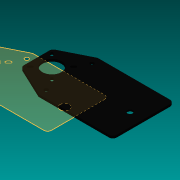
# Autodesk Inventor part: Y Slider
Saved by Autodesk Inventor 2016 (Build 200138000, 138)
## iProperties
Created: 2015-06-04
Part Number: Y Slider
Material: Aluminum 6061
Document SubType Name: Modeling
Designer: Sawaiz Syed
Density: 2.7 g/cm^3
Appearance: Anodized - Black
Author: Sawaiz Syed
Autodesk Inventor part; units mm, degrees
ref_plane "YZ Plane" through (0, 0, 0) normal (1, 0, 0) x (0, 1, 0)
ref_plane "XZ Plane" through (0, 0, 0) normal (0, 1, 0) x (-1, 0, 0)
ref_plane "XY Plane" through (0, 0, 0) normal (0, 0, 1) x (1, 0, 0)
sketch "Sketch1" plane through (0, 0, 0) normal (0, 0, 1) x (1, 0, 0)
  circle A0 centre (-2.41, 40.64) radius 12.5 projected
  line L0 (-16.506, 28.736) -> (-19.006, 26.236) projected
  arc A1 (-14.314, 26.544) -> (-16.506, 28.736) centre (-15.41, 27.64) ccw projected
  line L1 (-16.814, 24.044) -> (-14.314, 26.544) projected
  arc A2 (-19.006, 26.236) -> (-16.814, 24.044) centre (-17.91, 25.14) ccw projected
  line L2 (-19.006, 55.044) -> (-16.506, 52.544) projected
  arc A3 (-16.506, 52.544) -> (-14.314, 54.736) centre (-15.41, 53.64) ccw projected
  line L3 (-14.314, 54.736) -> (-16.814, 57.236) projected
  arc A4 (-16.814, 57.236) -> (-19.006, 55.044) centre (-17.91, 56.14) ccw projected
  line L4 (9.494, 26.544) -> (11.994, 24.044) projected
  arc A5 (11.686, 28.736) -> (9.494, 26.544) centre (10.59, 27.64) ccw projected
  line L5 (14.186, 26.236) -> (11.686, 28.736) projected
  arc A6 (11.994, 24.044) -> (14.186, 26.236) centre (13.09, 25.14) ccw projected
  line L6 (11.686, 52.544) -> (14.186, 55.044) projected
  arc A7 (9.494, 54.736) -> (11.686, 52.544) centre (10.59, 53.64) ccw projected
  line L7 (11.994, 57.236) -> (9.494, 54.736) projected
  arc A8 (14.186, 55.044) -> (11.994, 57.236) centre (13.09, 56.14) ccw projected
  circle A9 centre (20.14, 70.64) radius 2.5 projected
  circle A10 centre (20.14, 10.64) radius 2.5 projected
  circle A11 centre (100.14, 40.64) radius 3.57 projected
  line L8 (-22.41, 20.64) -> (-22.41, 60.64)
  line L9 (-22.41, 60.64) -> (17.59, 80.64)
  line L10 (17.59, 80.64) -> (117.59, 80.64)
  line L11 (117.59, 80.64) -> (117.59, 0.64)
  line L12 (117.59, 0.64) -> (20.14, 0.64)
  line L13 (20.14, 0.64) -> (-22.41, 20.64)
  point P0 (0, 0)
  dimension "d0" = 20
  dimension "d1" = 0
  dimension "d2" = 80
  dimension "d3" = 90
  dimension "d4" = 90
  dimension "d5" = 10
  dimension "d6" = 100
  dimension "d7" = 140
  dimension "d8" = 40
  dimension "d9" = 20
  constraints: 12 end point, 1 parallel, 1 vertical
  measures "d0" distance from line of L8 A0.centre
  measures "d1" horizontal distance of A10.centre L12.end
  measures "d2" distance of L10.end L11.end
  measures "d3" angle of L12 L11
  measures "d4" angle of L11 L10
  measures "d5" distance from line of L10 A9.centre
  measures "d6" distance of L9.end L10.end
  measures "d7" distance between parallel lines of L8 L11
  measures "d8" distance of L8.start L8.end
  measures "d9" horizontal distance of L8.start A0.centre
extrude "Extrusion1" add sketch "Sketch1" along normal blind 3
fillet "Fillet1" radius 5 6 edges at (117.59, 80.64, 1.5) (117.59, 0.64, 1.5) (17.59, 80.64, 1.5) (-22.41, 60.64, 1.5) (-22.41, 20.64, 1.5) (20.14, 0.64, 1.5)
sketch "Sketch2" plane through (0, 0, 0) normal (0, 0, -1) x (-1, 0, 0)
  circle A0 centre (2.41, 40.64) radius 12.5 projected
  circle A1 centre (-100.14, 40.64) radius 3.57 projected
  circle A2 centre (-20.14, 10.64) radius 2.5 projected
  circle A3 centre (-20.14, 70.64) radius 2.5 projected
  arc A4 (-11.686, 52.544) -> (-9.494, 54.736) centre (-10.59, 53.64) ccw projected
  line L0 (-11.686, 52.544) -> (-14.186, 55.044) projected
  arc A5 (-11.994, 57.236) -> (-14.186, 55.044) centre (-13.09, 56.14) ccw projected
  line L1 (-11.994, 57.236) -> (-9.494, 54.736) projected
  arc A6 (-9.494, 26.544) -> (-11.686, 28.736) centre (-10.59, 27.64) ccw projected
  line L2 (-9.494, 26.544) -> (-11.994, 24.044) projected
  arc A7 (-14.186, 26.236) -> (-11.994, 24.044) centre (-13.09, 25.14) ccw projected
  line L3 (-14.186, 26.236) -> (-11.686, 28.736) projected
  arc A8 (19.006, 55.044) -> (16.814, 57.236) centre (17.91, 56.14) ccw projected
  line L4 (19.006, 55.044) -> (16.506, 52.544) projected
  arc A9 (14.314, 54.736) -> (16.506, 52.544) centre (15.41, 53.64) ccw projected
  line L5 (14.314, 54.736) -> (16.814, 57.236) projected
  arc A10 (16.506, 28.736) -> (14.314, 26.544) centre (15.41, 27.64) ccw projected
  line L6 (16.506, 28.736) -> (19.006, 26.236) projected
  arc A11 (16.814, 24.044) -> (19.006, 26.236) centre (17.91, 25.14) ccw projected
  line L7 (16.814, 24.044) -> (14.314, 26.544) projected
  arc A12 (-21.2565, 0.64) -> (-19.1296, 1.1149) centre (-21.2565, 5.64) ccw projected
  line L8 (-19.1296, 1.1149) -> (19.5369, 19.2896) projected
  arc A13 (19.5369, 19.2896) -> (22.41, 23.8146) centre (17.41, 23.8146) ccw projected
  line L9 (22.41, 23.8146) -> (22.41, 57.5498) projected
  arc A14 (22.41, 57.5498) -> (19.6461, 62.022) centre (17.41, 57.5498) ccw projected
  line L10 (19.6461, 62.022) -> (-16.5343, 80.1121) projected
  arc A15 (-16.5343, 80.1121) -> (-18.7703, 80.64) centre (-18.7703, 75.64) ccw projected
  line L11 (-18.7703, 80.64) -> (-112.59, 80.64) projected
  arc A16 (-112.59, 80.64) -> (-117.59, 75.64) centre (-112.59, 75.64) ccw projected
  line L12 (-117.59, 75.64) -> (-117.59, 5.64) projected
  arc A17 (-117.59, 5.64) -> (-112.59, 0.64) centre (-112.59, 5.64) ccw projected
  line L13 (-112.59, 0.64) -> (-21.2565, 0.64) projected
  point P0 (0, 0)
  constraints: 1 coincident
hole "Hole1" at (100.14, 40.64, 0) direction (0, 0, 1) diameter 12 depth 1
sketch "Sketch3" plane through (0, 0, 0) normal (0, 0, -1) x (-1, 0, 0)
  circle A0 centre (-20.14, 10.64) radius 2.5 projected
  circle A1 centre (-100.14, 40.64) radius 6 projected
  circle A2 centre (2.41, 40.64) radius 12.5 projected
  circle A3 centre (-20.14, 10.64) radius 2.5 projected
  circle A4 centre (-20.14, 70.64) radius 2.5 projected
  arc A5 (-11.686, 52.544) -> (-9.494, 54.736) centre (-10.59, 53.64) ccw projected
  line L0 (-11.686, 52.544) -> (-14.186, 55.044) projected
  arc A6 (-11.994, 57.236) -> (-14.186, 55.044) centre (-13.09, 56.14) ccw projected
  line L1 (-11.994, 57.236) -> (-9.494, 54.736) projected
  arc A7 (-9.494, 26.544) -> (-11.686, 28.736) centre (-10.59, 27.64) ccw projected
  line L2 (-9.494, 26.544) -> (-11.994, 24.044) projected
  arc A8 (-14.186, 26.236) -> (-11.994, 24.044) centre (-13.09, 25.14) ccw projected
  line L3 (-14.186, 26.236) -> (-11.686, 28.736) projected
  arc A9 (19.006, 55.044) -> (16.814, 57.236) centre (17.91, 56.14) ccw projected
  line L4 (19.006, 55.044) -> (16.506, 52.544) projected
  arc A10 (14.314, 54.736) -> (16.506, 52.544) centre (15.41, 53.64) ccw projected
  line L5 (14.314, 54.736) -> (16.814, 57.236) projected
  arc A11 (16.506, 28.736) -> (14.314, 26.544) centre (15.41, 27.64) ccw projected
  line L6 (16.506, 28.736) -> (19.006, 26.236) projected
  arc A12 (16.814, 24.044) -> (19.006, 26.236) centre (17.91, 25.14) ccw projected
  line L7 (16.814, 24.044) -> (14.314, 26.544) projected
  arc A13 (-21.2565, 0.64) -> (-19.1296, 1.1149) centre (-21.2565, 5.64) ccw projected
  line L8 (-19.1296, 1.1149) -> (19.5369, 19.2896) projected
  arc A14 (19.5369, 19.2896) -> (22.41, 23.8146) centre (17.41, 23.8146) ccw projected
  line L9 (22.41, 23.8146) -> (22.41, 57.5498) projected
  arc A15 (22.41, 57.5498) -> (19.6461, 62.022) centre (17.41, 57.5498) ccw projected
  line L10 (19.6461, 62.022) -> (-16.5343, 80.1121) projected
  arc A16 (-16.5343, 80.1121) -> (-18.7703, 80.64) centre (-18.7703, 75.64) ccw projected
  line L11 (-18.7703, 80.64) -> (-112.59, 80.64) projected
  arc A17 (-112.59, 80.64) -> (-117.59, 75.64) centre (-112.59, 75.64) ccw projected
  line L12 (-117.59, 75.64) -> (-117.59, 5.64) projected
  arc A18 (-117.59, 5.64) -> (-112.59, 0.64) centre (-112.59, 5.64) ccw projected
  line L13 (-112.59, 0.64) -> (-21.2565, 0.64) projected
  circle A19 centre (-20.14, 70.64) radius 2.0572 projected
  circle A20 centre (-20.14, 10.64) radius 2.0572 projected
  point P0 (0, 0)
  constraints: 2 coincident
hole "Hole2" at (20.14, 10.64, 0) at (20.14, 70.64, 0) direction (0, 0, 1) diameter 8.1 depth 1
body "Solid1"
